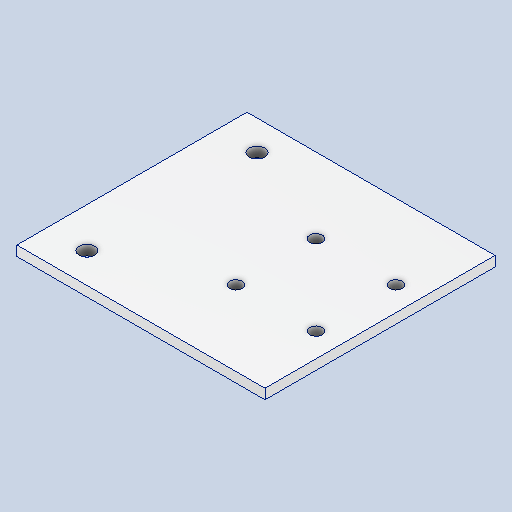
# Autodesk Inventor part: MotorMount
Saved by Autodesk Inventor 2023 (Build 270158000, 158)
## iProperties
Created: 2022-09-11
Part Number: MotorMount
Material: Aluminum 6061
Document SubType Name: Modeling
Designer: PC
Density: 2.7 g/cm^3
Appearance: Aluminum - Flat
Mass: 48.5159 g
Surface Area: 125.435 cm^2
Volume: 17.9688 cm^3
Author: PC
Autodesk Inventor part; units mm, degrees
ref_plane "YZ Plane" through (0, 0, 0) normal (1, 0, 0) x (0, 1, 0)
ref_plane "XZ Plane" through (0, 0, 0) normal (0, 1, 0) x (-1, 0, 0)
ref_plane "XY Plane" through (0, 0, 0) normal (0, 0, 1) x (1, 0, 0)
sketch "Sketch1" plane through (0, 0, 0) normal (0, 1, 0) x (-1, 0, 0)
  line L0 (0, 0) -> (101.6, 0)
  line L1 (101.6, 0) -> (101.6, -47.625)
  line L2 (101.6, -47.625) -> (0, -47.625)
  line L3 (0, -47.625) -> (0, 0)
  circle A0 centre (88.9, -9.525) radius 2.5
  circle A1 centre (88.9, -38.1) radius 2.5
  circle A2 centre (7.62, -11.1125) radius 2.0193
  circle A3 centre (33.02, -11.1125) radius 2.0193
  circle A4 centre (33.02, -36.5125) radius 2.0193
  circle A5 centre (7.62, -36.5125) radius 2.0193
  line L4 (0, 0) -> (0, -40.7836)
  point P0 (37.1991, -51.2989)
  point P1 (24.9809, -31.7225)
  point P2 (38.4109, -31.7225)
  dimension "d0" = 101.6
  dimension "d1" = 47.625
  dimension "d2" = 5
  dimension "d3" = 5
  dimension "d4" = 12.7
  dimension "d5" = 12.7
  dimension "d6" = 9.525
  dimension "d7" = 9.525
  dimension "d8" = 25.4
  dimension "d9" = 25.4
  dimension "d10" = 25.4
  dimension "d11" = 25.4
  dimension "d12" = 4.0386
  dimension "d13" = 4.0386
  dimension "d14" = 4.0386
  dimension "d15" = 4.0386
  dimension "d16" = 11.1125
  constraints: 10 end point, 6 centre point, 2 parallel, 1 horizontal, 1 perpendicular
  measures "d0" distance of L1.end L2.end
  measures "d1" distance of L0.end L1.end
  measures "d2" diameter of A0
  measures "d3" diameter of A1
  measures "d4" distance from line of L1 A0.centre
  measures "d5" distance from line of L1 A1.centre
  measures "d6" distance from line of L0 A0.centre
  measures "d7" distance from line of L2 A1.centre
  measures "d8" distance of A4.centre A3.centre
  measures "d9" distance of A2.centre A3.centre
  measures "d10" distance of A5.centre A2.centre
  measures "d11" distance of A4.centre A5.centre
  measures "d12" diameter of A2
  measures "d13" diameter of A3
  measures "d14" diameter of A4
  measures "d15" diameter of A5
  measures "d16" distance from line of L0 A2.centre
extrude "Extrusion1" add sketch "Sketch1" along normal blind 3.175
sketch "Sketch2" plane through (0, 3.175, 0) normal (0, 1, 0) x (1, 0, 0)
  line L0 (-101.6, 47.625) -> (-101.6, 0) projected
  line L1 (-101.6, 0) -> (0, 0) projected
  line L2 (0, 0) -> (0, 47.625) projected
  line L3 (0, 47.625) -> (-101.6, 47.625) projected
  circle A0 centre (-88.9, 9.525) radius 2.5 projected
  circle A1 centre (-88.9, 38.1) radius 2.5 projected
  circle A2 centre (-7.62, 11.1125) radius 2.0193 projected
  circle A3 centre (-33.02, 11.1125) radius 2.0193 projected
  circle A4 centre (-33.02, 36.5125) radius 2.0193 projected
  circle A5 centre (-7.62, 36.5125) radius 2.0193 projected
  line L4 (-78.74, 0) -> (-78.74, 47.625)
  line L5 (0, 47.625) -> (-101.6, 47.625) projected
  line L6 (0, -12.7) -> (-78.74, -12.7)
  line L7 (-78.74, -12.7) -> (-78.74, 60.325)
  line L8 (-78.74, 60.325) -> (0, 60.325)
  line L9 (0, 60.325) -> (0, -12.7)
  circle A6 centre (-66.04, -3.175) radius 2.5
  circle A7 centre (-66.04, 50.8) radius 2.5
  dimension "d19" = 78.74
  dimension "d20" = 9.525
  dimension "d21" = 12.7
  dimension "d22" = 12.7
  dimension "d23" = 9.525
  dimension "d24" = 12.7
  dimension "d25" = 12.7
  constraints: 10 end point, 2 centre point, 2 parallel, 2 perpendicular, 2 point on line, 1 horizontal
  measures "d19" distance between parallel lines of L2 L4
  measures "d20" distance from line of L8 A7.centre
  measures "d21" distance from line of L7 A7.centre
  measures "d22" distance from line of L7 A6.centre
  measures "d23" distance from line of L6 A6.centre
  measures "d24" distance between parallel lines of L3 L8
  measures "d25" distance between parallel lines of L1 L6
extrude "Extrusion2" add sketch "Sketch2" against normal blind 3.175 contours L7 L8 L9 L3 | L3 L2 L1 L4 | L1 L9 L6 L7
extrude "Extrusion3" cut sketch "Sketch2" against normal through all contours L3 L4 L1 L0
equation "\"d5\" = d4"
equation "\"d6\" = 0.2 * d1"
equation "\"d7\" = d6"
equation "\"d20\" = d7"
equation "\"d21\" = d5"
equation "\"d23\" = d20"
equation "\"d25\" = d24"
body "Solid1"
